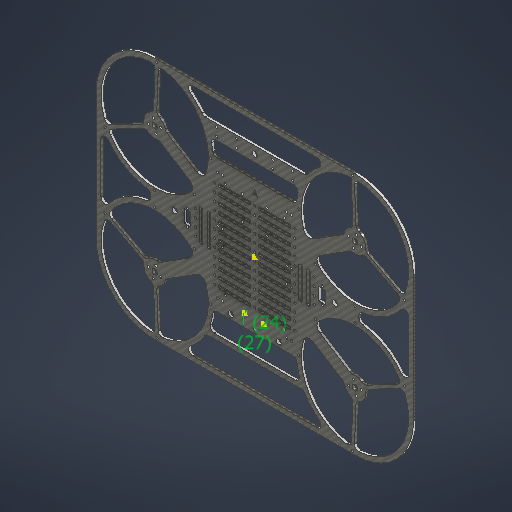
# Autodesk Inventor part: v3_bottom_carbon_fiber
Saved by Autodesk Inventor 2026 (Build 300175050, 175E)
## iProperties
Created: 2025-03-06
Part Number: v3_bottom_carbon_fiber
Material: Generic
Document SubType Name: Modeling
Designer: Bruno
Density: 1 g/cm^3
Appearance: Default
Author: Bruno
Autodesk Inventor part; units mm, degrees
ref_plane "YZ Plane" through (0, 0, 0) normal (1, 0, 0) x (0, 1, 0)
ref_plane "XZ Plane" through (0, 0, 0) normal (0, 1, 0) x (-1, 0, 0)
ref_plane "XY Plane" through (0, 0, 0) normal (0, 0, 1) x (1, 0, 0)
sketch "Sketch1" plane through (0, 0, 0) normal (0, 0, 1) x (1, 0, 0)
  line L0 (-125, 79) -> (125, 79)
  line L1 (-125, 79) -> (-125, -79)
  line L2 (-125, -79) -> (125, -79)
  line L3 (125, -79) -> (125, 79)
  line L4 (-234.9943, 0) -> (246.4628, 0)
  line L5 (0, 171.5298) -> (0, -171.5298)
  line L6 (52.1097, 83) -> (0, 83)
  line L7 (130, 6.1714) -> (130, 0)
  line L8 (198, 79) -> (198, 0)
  line L9 (125, 152) -> (0, 152)
  line L10 (52.1097, -83) -> (0, -83)
  line L11 (130, -6.1714) -> (130, 0)
  line L12 (198, -79) -> (198, 0)
  line L13 (125, -152) -> (0, -152)
  line L14 (125, 146) -> (0, 146)
  line L15 (192, 79) -> (192, 0)
  line L16 (125, -146) -> (0, -146)
  line L17 (192, -79) -> (192, 0)
  line L18 (-52.1097, 83) -> (0, 83)
  line L19 (-130, 6.1714) -> (-130, 0)
  line L20 (-198, 79) -> (-198, 0)
  line L21 (-125, 152) -> (0, 152)
  line L22 (-125, -152) -> (0, -152)
  line L23 (-52.1097, -83) -> (0, -83)
  line L24 (-198, -79) -> (-198, 0)
  line L25 (-130, -6.1714) -> (-130, 0)
  line L26 (-125, 146) -> (0, 146)
  line L27 (-192, 79) -> (-192, 0)
  line L28 (-125, -146) -> (0, -146)
  line L29 (-192, -79) -> (-192, 0)
  circle A0 centre (122.1995, 148.944) radius 1.5
  circle A1 centre (186.9735, 46.4534) radius 1.5
  circle A2 centre (125, 9) radius 1.5
  circle A3 centre (55, 79) radius 1.5
  circle A4 centre (75.5025, 29.5025) radius 1.5
  circle A5 centre (122.1995, -148.944) radius 1.5
  circle A6 centre (186.9735, -46.4534) radius 1.5
  circle A7 centre (125, -9) radius 1.5
  circle A8 centre (55, -79) radius 1.5
  circle A9 centre (75.5025, -29.5025) radius 1.5
  circle A10 centre (-122.1995, 148.944) radius 1.5
  circle A11 centre (-186.9735, 46.4534) radius 1.5
  circle A12 centre (-125, 9) radius 1.5
  circle A13 centre (-55, 79) radius 1.5
  circle A14 centre (-75.5025, 29.5025) radius 1.5
  circle A15 centre (-122.1995, -148.944) radius 1.5
  circle A16 centre (-55, -79) radius 1.5
  circle A17 centre (-75.5025, -29.5025) radius 1.5
  circle A18 centre (-125, -9) radius 1.5
  circle A19 centre (-186.9735, -46.4534) radius 1.5
  line L30 (-125, -79) -> (125, 79)
  line L31 (75.5025, 29.5025) -> (125, 79)
  line L32 (122.1995, 148.944) -> (125, 79)
  line L33 (125, 79) -> (186.9735, 46.4534)
  circle A20 centre (125, 79) radius 70
  circle A21 centre (125, 79) radius 13.5
  circle A22 centre (125, 79) radius 3.5
  circle A23 centre (125, 79) radius 8
  line L34 (120.0816, 66.4278) -> (73.0422, 36.6989)
  line L35 (111.5337, 79.9531) -> (64.4942, 50.2241)
  line L36 (126.4643, 92.4204) -> (124.3191, 145.9965)
  line L37 (135.8902, 71.0217) -> (183.3612, 46.0914)
  line L38 (122.4675, 92.2603) -> (120.3223, 145.8365)
  line L39 (137.7501, 74.5631) -> (185.221, 49.6328)
  circle A24 centre (125, -79) radius 13.5
  circle A25 centre (125, -79) radius 3.5
  line L40 (120.0816, -66.4278) -> (73.0422, -36.6989)
  line L41 (111.5337, -79.9531) -> (64.4942, -50.2241)
  line L42 (126.4643, -92.4204) -> (124.3191, -145.9965)
  line L43 (135.8902, -71.0217) -> (183.3612, -46.0914)
  line L44 (122.4675, -92.2603) -> (120.3223, -145.8365)
  line L45 (137.7501, -74.5631) -> (185.221, -49.6328)
  circle A26 centre (-125, 79) radius 13.5
  circle A27 centre (-125, 79) radius 3.5
  line L46 (-120.0816, 66.4278) -> (-73.0422, 36.6989)
  line L47 (-111.5337, 79.9531) -> (-64.4942, 50.2241)
  line L48 (-126.4643, 92.4204) -> (-124.3191, 145.9965)
  line L49 (-135.8902, 71.0217) -> (-183.3612, 46.0914)
  line L50 (-122.4675, 92.2603) -> (-120.3223, 145.8365)
  line L51 (-137.7501, 74.5631) -> (-185.221, 49.6328)
  circle A28 centre (-125, -79) radius 13.5
  circle A29 centre (-125, -79) radius 3.5
  line L52 (-137.7501, -74.5631) -> (-185.221, -49.6328)
  line L53 (-135.8902, -71.0217) -> (-183.3612, -46.0914)
  line L54 (-120.0816, -66.4278) -> (-73.0422, -36.6989)
  line L55 (-111.5337, -79.9531) -> (-64.4942, -50.2241)
  line L56 (-122.4675, -92.2603) -> (-120.3223, -145.8365)
  line L57 (-126.4643, -92.4204) -> (-124.3191, -145.9965)
  circle A30 centre (125, 79) radius 67
  circle A31 centre (125, 79) radius 73
  circle A32 centre (125, -79) radius 67
  circle A33 centre (125, -79) radius 73
  circle A34 centre (-125, 79) radius 67
  circle A35 centre (-125, 79) radius 73
  circle A36 centre (-125, -79) radius 67
  circle A37 centre (-125, -79) radius 73
  circle A38 centre (117.1959, 80.7597) radius 1.5
  line L58 (117.1959, 80.7597) -> (125, 79)
  circle A39 centre (123.2403, 71.1959) radius 1.5
  circle A40 centre (132.8041, 77.2403) radius 1.5
  circle A41 centre (126.7597, 86.8041) radius 1.5
  circle A42 centre (117.1959, -80.7597) radius 1.5
  circle A43 centre (123.2403, -71.1959) radius 1.5
  circle A44 centre (132.8041, -77.2403) radius 1.5
  circle A45 centre (126.7597, -86.8041) radius 1.5
  circle A46 centre (-117.1959, 80.7597) radius 1.5
  circle A47 centre (-123.2403, 71.1959) radius 1.5
  circle A48 centre (-132.8041, 77.2403) radius 1.5
  circle A49 centre (-126.7597, 86.8041) radius 1.5
  circle A50 centre (-117.1959, -80.7597) radius 1.5
  circle A51 centre (-126.7597, -86.8041) radius 1.5
  circle A52 centre (-123.2403, -71.1959) radius 1.5
  circle A53 centre (-132.8041, -77.2403) radius 1.5
  point P0 (0, 0)
  point P1 (-125, 0)
  point P2 (125, 0)
  point P3 (0, 79)
  point P4 (0, 0)
  point P5 (111.5337, 79.9531)
  point P6 (-111.5337, 79.9531)
  point P7 (-122.4675, 92.2603)
  point P8 (-137.7501, -74.5631)
  point P9 (-122.4675, -92.2603)
  point P10 (-111.5337, -79.9531)
  point P11 (111.5337, -79.9531)
  point P12 (122.4675, -92.2603)
  point P13 (137.7501, -74.5631)
  point P14 (73.0422, 36.6989)
  point P15 (115.6927, 140.8593)
  point P16 (122.3195, 145.9464)
  point P17 (122.3173, 146)
  point P18 (120, 141)
  point P19 (192, 50.0172)
  point P20 (192, -50.0172)
  point P21 (-125, 152)
  point P22 (-198, 79)
  point P23 (-198, -79)
  point P24 (-125, -152)
  point P25 (125, -152)
  point P26 (198, -79)
  point P27 (96.0172, 146)
  point P28 (-96.0172, 146)
  point P29 (52.1097, -83)
  point P30 (96.0172, -146)
  point P31 (-96.0172, -146)
  point P32 (-52.1097, -83)
  point P33 (-183.3612, 46.0914)
  point P34 (-119.6903, 140.9993)
  point P35 (-192, -50.0172)
  point P36 (-192, 50.0172)
  point P37 (-130, -6.1714)
  point P38 (-73.0422, -36.6989)
  point P39 (-120.3223, -145.8365)
  point P40 (-119.6903, -140.9993)
  point P41 (-185.221, -49.6328)
  point P42 (-183.3612, -46.0914)
  point P43 (64.4942, -50.2241)
  point P44 (73.0422, -36.6989)
  point P45 (124.3191, -145.9965)
  point P46 (120.3223, -145.8365)
  point P47 (124.4599, 92.4892)
  point P48 (68.363, 43.2054)
  point P49 (113.5881, 71.7877)
  dimension "d71" = 16
  dimension "d2" = 250
  dimension "d3" = 158
  dimension "d16" = 166
  dimension "d17" = 260
  dimension "d35" = 3
  dimension "d36" = 3
  dimension "d37" = 3
  dimension "d40" = 3
  dimension "d42" = 3
  dimension "d62" = 45
  dimension "d64" = 120
  dimension "d65" = 120
  dimension "d66" = 140
  dimension "d67" = 27
  dimension "d68" = 7
  dimension "d76" = 16
  dimension "d77" = 4
  dimension "d78" = 4
  dimension "d95" = 32.293
  dimension "d150" = 134
  dimension "d151" = 146
  dimension "d158" = 3
  dimension "d159" = 45
  dimension "d162" = 360
  dimension "d168" = 6
  constraints: 118 end point, 100 symmetric about line, 53 centre point, 31 point on circle, 14 coincident, 11 point on line, 7 perpendicular, 6 parallel, 6 tangent, 4 midpoint, 3 horizontal, 1 vertical, 51 other
  measures "d2" distance of L0.start L0.end
  measures "d3" distance of L2.end L0.end
  measures "d16" diameter of L6 L4
  measures "d17" diameter of L7 L5
  measures "d35" diameter of A0
  measures "d36" diameter of A1
  measures "d37" diameter of A2
  measures "d40" diameter of A3
  measures "d42" diameter of A4
  measures "d62" angle of L0 L31
  measures "d64" angle of L30 L33
  measures "d65" angle of L30 L32
  measures "d66" diameter of A20
  measures "d67" diameter of A21
  measures "d68" diameter of A22
  measures "d76" diameter of L34 L30
  measures "d77" diameter of L36 L32
  measures "d78" diameter of L37 L33
  measures "d95" angle of L30 L0
  measures "d150" diameter of A30
  measures "d151" diameter of A31
  measures "d158" diameter of A38
  measures "d159" angle of L30 L58
  measures "d168" radial gap between concentric circles of A31 A30
extrude "Extrusion1" add sketch "Sketch1" along normal blind 3 contours A27 L1 A26 L0 | L0 A26 L1 A27 | A26 L47 L0 | L0 L47 A34 L46 A26 | A34 L0 A13 A35 L1 A12 | L1 A12 A35 L27 A34 | L49 A34 L51 A26 | A34 L26 A35 L0 A13 | A26 L48 A34 L50 | A35 L0 L5 L4 L1 | L1 L4 L19 A35 | L27 A35 L26 A34 | A35 L18 L5 L0 | L4 L30 A37 L1 | L1 A37 L25 L4 | L27 L4 L20 A35 | L5 L6 A31 L0 | L0 A31 L30 L5 | A35 L21 L5 L26 | A37 L30 A36 L1 A18 | L1 A18 A36 L29 A37 | L30 A31 L3 L4 | L4 L3 A33 L2 L5 | L5 L2 A37 L30 | L29 A37 L24 L4 | A31 L14 A20 A3 L0 | L0 A3 A20 L30 A31 | L5 L9 A31 L14 | A37 L2 A16 A36 L30 | L4 L11 A33 L3 | L3 A31 L7 L4 | L5 L23 A37 L2 | L2 A33 L10 L5 | L30 A20 A4 A2 L3 A31 | L29 A36 L28 A37 | A31 L15 A20 A0 L14 | A36 L55 L2 A28 L30 | L30 A28 L54 A36 | A37 L28 A36 L2 A16 | A33 L17 A32 L3 A7 | L3 A7 A32 L2 A8 A33 | L3 A2 A20 A1 L15 A31 | L2 A8 A32 L16 A33 | A20 A3 L0 A30 L30 | L30 A30 L31 A4 A20 | A20 L14 L32 A30 L0 A3 | A20 A0 L32 L14 | A28 L2 A29 L30 | L30 A29 L1 A28 | L15 A31 L8 L4 | L4 L12 A33 L17 | L16 A33 L13 L5 | L5 L22 A37 L28 | A30 L35 L0 A21 L30 | L30 A21 L31 L34 A30 | A36 L53 A28 L52 | L32 A0 A20 L15 A30 L14 | L14 A30 L32 | L1 A29 L2 A28 | L2 L55 A28 | A33 L16 A32 L17 | A20 A4 L31 A30 L3 A2 | A21 L0 A23 L30 | L30 A23 L31 A21 | L57 A28 L56 A36 | A30 L36 A21 L32 | L32 A21 L38 A30 | L3 A30 L33 A1 A20 A2 | A20 A1 L33 A30 L15 | A23 L0 A22 L30 | L30 A22 L31 A23 | A21 L32 A23 A38 L0 | L0 L35 A21 | A21 L34 L31 | L31 A23 A39 L3 A21 | A21 L33 A23 A40 A41 L32 | A24 L2 A25 L3 | L3 A25 L2 A24 | A32 L45 A24 L43 | L40 A24 L2 L41 A32 | L2 A24 L41 | L44 A24 L42 A32 | A23 A38 L58 A22 L0 | L31 A22 L3 A23 A39 | A30 L33 A21 L39 | A23 A41 A40 L33 A22 L32 | L32 A22 L58 A38 A23 | L3 A23 L33 A21 | L37 A21 L33 A30 | L3 A22 L33 A23
fillet "Fillet1" radius 5 47 edges at (-130, 6.1714, 1.5) (-52.1097, 83, 1.5) (-135.8902, 71.0217, 1.5) (-122.4675, 92.2603, 1.5) (-126.4643, 92.4204, 1.5) (-137.7501, 74.5631, 1.5) (-137.7501, -74.5631, 1.5) (-135.8902, -71.0217, 1.5) (-126.4643, -92.4204, 1.5) (-122.4675, -92.2603, 1.5) (126.4643, -92.4204, 1.5) (122.4675, -92.2603, 1.5) (137.7501, -74.5631, 1.5) (135.8902, -71.0217, 1.5) (137.7501, 74.5631, 1.5) (135.8902, 71.0217, 1.5) (126.4643, 92.4204, 1.5) (122.4675, 92.2603, 1.5) (-120.3223, 145.8365, 1.5) (-183.3612, 46.0914, 1.5) (-185.221, 49.6328, 1.5) (-192, 50.0172, 1.5) (-96.0172, 146, 1.5) (-130, -6.1714, 1.5) (-192, -50.0172, 1.5) (-185.221, -49.6328, 1.5) (-183.3612, -46.0914, 1.5) (-120.3223, -145.8365, 1.5) (-96.0172, -146, 1.5) (-52.1097, -83, 1.5) (52.1097, -83, 1.5) (96.0172, -146, 1.5) (120.3223, -145.8365, 1.5) (124.3191, -145.9965, 1.5) (192, -50.0172, 1.5) (185.221, -49.6328, 1.5) (183.3612, -46.0914, 1.5) (130, -6.1714, 1.5) (130, 6.1714, 1.5) (192, 50.0172, 1.5) (185.221, 49.6328, 1.5) (183.3612, 46.0914, 1.5) (124.3191, 145.9965, 1.5) (96.0172, 146, 1.5) (52.1097, 83, 1.5) (-124.3191, 145.9965, 1.5) (-124.3191, -145.9965, 1.5)
fillet "Fillet2" radius 5 8 edges at (120.0816, 66.4278, 1.5) (111.5337, 79.9531, 1.5) (120.0816, -66.4278, 1.5) (111.5337, -79.9531, 1.5) (-111.5337, -79.9531, 1.5) (-120.0816, -66.4278, 1.5) (-111.5337, 79.9531, 1.5) (-120.0816, 66.4278, 1.5)
fillet "Fillet3" radius 8 8 edges at (64.4942, -50.2241, 1.5) (73.0422, -36.6989, 1.5) (64.4942, 50.2241, 1.5) (73.0422, 36.6989, 1.5) (-64.4942, 50.2241, 1.5) (-73.0422, 36.6989, 1.5) (-73.0422, -36.6989, 1.5) (-64.4942, -50.2241, 1.5)
sketch "Sketch2" plane through (0, 0, 3) normal (0, 0, 1) x (1, 0, 0)
  line L0 (-253.4929, 0) -> (253.4929, 0)
  line L1 (0, 210.0752) -> (0, -210.0752)
  line L2 (-46, -68) -> (46, -68)
  line L3 (46, -68) -> (46, -10)
  line L4 (46, -10) -> (-46, -10)
  line L5 (-46, -10) -> (-46, -68)
  circle A0 centre (-46, -68) radius 1.5
  circle A1 centre (46, -68) radius 1.5
  circle A2 centre (46, -10) radius 1.5
  circle A3 centre (-46, -10) radius 1.5
  line L6 (-47.521, -83) -> (47.521, -83) projected
  line L7 (-44, -53) -> (-6, -53)
  line L8 (-5, -54) -> (-5, -56)
  line L9 (-6, -57) -> (-44, -57)
  line L10 (-45, -56) -> (-45, -54)
  circle A4 centre (0, -55) radius 1.5
  line L11 (-59.788, -55) -> (59.788, -55)
  circle A5 centre (-50, -55) radius 1.5
  arc A6 (-45, -56) -> (-44, -57) centre (-44, -56) ccw
  arc A7 (-44, -53) -> (-45, -54) centre (-44, -54) ccw
  arc A8 (-6, -57) -> (-5, -56) centre (-6, -56) ccw
  arc A9 (-5, -54) -> (-6, -53) centre (-6, -54) ccw
  line L12 (44, -53) -> (6, -53)
  line L13 (5, -54) -> (5, -56)
  line L14 (6, -57) -> (44, -57)
  line L15 (45, -56) -> (45, -54)
  circle A10 centre (50, -55) radius 1.5
  arc A11 (44, -57) -> (45, -56) centre (44, -56) ccw
  arc A12 (45, -54) -> (44, -53) centre (44, -54) ccw
  arc A13 (5, -56) -> (6, -57) centre (6, -56) ccw
  arc A14 (6, -53) -> (5, -54) centre (6, -54) ccw
  circle A15 centre (-50, -45) radius 1.5
  line L16 (-45, -46) -> (-45, -44)
  arc A16 (-44, -43) -> (-45, -44) centre (-44, -44) ccw
  line L17 (-44, -43) -> (-6, -43)
  arc A17 (-45, -46) -> (-44, -47) centre (-44, -46) ccw
  line L18 (-6, -47) -> (-44, -47)
  arc A18 (-5, -44) -> (-6, -43) centre (-6, -44) ccw
  line L19 (-5, -44) -> (-5, -46)
  arc A19 (-6, -47) -> (-5, -46) centre (-6, -46) ccw
  circle A20 centre (0, -45) radius 1.5
  line L20 (5, -44) -> (5, -46)
  arc A21 (6, -43) -> (5, -44) centre (6, -44) ccw
  line L21 (44, -43) -> (6, -43)
  arc A22 (5, -46) -> (6, -47) centre (6, -46) ccw
  line L22 (6, -47) -> (44, -47)
  arc A23 (44, -47) -> (45, -46) centre (44, -46) ccw
  line L23 (45, -46) -> (45, -44)
  arc A24 (45, -44) -> (44, -43) centre (44, -44) ccw
  circle A25 centre (50, -45) radius 1.5
  circle A26 centre (-50, -35) radius 1.5
  line L24 (-45, -36) -> (-45, -34)
  arc A27 (-44, -33) -> (-45, -34) centre (-44, -34) ccw
  line L25 (-44, -33) -> (-6, -33)
  arc A28 (-45, -36) -> (-44, -37) centre (-44, -36) ccw
  line L26 (-6, -37) -> (-44, -37)
  arc A29 (-5, -34) -> (-6, -33) centre (-6, -34) ccw
  line L27 (-5, -34) -> (-5, -36)
  arc A30 (-6, -37) -> (-5, -36) centre (-6, -36) ccw
  circle A31 centre (0, -35) radius 1.5
  line L28 (5, -34) -> (5, -36)
  arc A32 (6, -33) -> (5, -34) centre (6, -34) ccw
  line L29 (44, -33) -> (6, -33)
  arc A33 (5, -36) -> (6, -37) centre (6, -36) ccw
  line L30 (6, -37) -> (44, -37)
  arc A34 (44, -37) -> (45, -36) centre (44, -36) ccw
  line L31 (45, -36) -> (45, -34)
  arc A35 (45, -34) -> (44, -33) centre (44, -34) ccw
  circle A36 centre (50, -35) radius 1.5
  circle A37 centre (-50, -25) radius 1.5
  line L32 (-45, -26) -> (-45, -24)
  arc A38 (-44, -23) -> (-45, -24) centre (-44, -24) ccw
  line L33 (-44, -23) -> (-6, -23)
  arc A39 (-45, -26) -> (-44, -27) centre (-44, -26) ccw
  line L34 (-6, -27) -> (-44, -27)
  arc A40 (-5, -24) -> (-6, -23) centre (-6, -24) ccw
  line L35 (-5, -24) -> (-5, -26)
  arc A41 (-6, -27) -> (-5, -26) centre (-6, -26) ccw
  circle A42 centre (0, -25) radius 1.5
  line L36 (5, -24) -> (5, -26)
  arc A43 (6, -23) -> (5, -24) centre (6, -24) ccw
  line L37 (44, -23) -> (6, -23)
  arc A44 (5, -26) -> (6, -27) centre (6, -26) ccw
  line L38 (6, -27) -> (44, -27)
  arc A45 (44, -27) -> (45, -26) centre (44, -26) ccw
  line L39 (45, -26) -> (45, -24)
  arc A46 (45, -24) -> (44, -23) centre (44, -24) ccw
  circle A47 centre (50, -25) radius 1.5
  circle A48 centre (-50, -15) radius 1.5
  line L40 (-45, -16) -> (-45, -14)
  arc A49 (-44, -13) -> (-45, -14) centre (-44, -14) ccw
  line L41 (-44, -13) -> (-6, -13)
  arc A50 (-45, -16) -> (-44, -17) centre (-44, -16) ccw
  line L42 (-6, -17) -> (-44, -17)
  arc A51 (-5, -14) -> (-6, -13) centre (-6, -14) ccw
  line L43 (-5, -14) -> (-5, -16)
  arc A52 (-6, -17) -> (-5, -16) centre (-6, -16) ccw
  circle A53 centre (0, -15) radius 1.5
  line L44 (5, -14) -> (5, -16)
  arc A54 (6, -13) -> (5, -14) centre (6, -14) ccw
  line L45 (44, -13) -> (6, -13)
  arc A55 (5, -16) -> (6, -17) centre (6, -16) ccw
  line L46 (6, -17) -> (44, -17)
  arc A56 (44, -17) -> (45, -16) centre (44, -16) ccw
  line L47 (45, -16) -> (45, -14)
  arc A57 (45, -14) -> (44, -13) centre (44, -14) ccw
  circle A58 centre (50, -15) radius 1.5
  circle A59 centre (-50, -5) radius 1.5
  line L48 (-45, -6) -> (-45, -4)
  arc A60 (-44, -3) -> (-45, -4) centre (-44, -4) ccw
  line L49 (-44, -3) -> (-6, -3)
  arc A61 (-45, -6) -> (-44, -7) centre (-44, -6) ccw
  line L50 (-6, -7) -> (-44, -7)
  arc A62 (-5, -4) -> (-6, -3) centre (-6, -4) ccw
  line L51 (-5, -4) -> (-5, -6)
  arc A63 (-6, -7) -> (-5, -6) centre (-6, -6) ccw
  circle A64 centre (0, -5) radius 1.5
  line L52 (5, -4) -> (5, -6)
  arc A65 (6, -3) -> (5, -4) centre (6, -4) ccw
  line L53 (44, -3) -> (6, -3)
  arc A66 (5, -6) -> (6, -7) centre (6, -6) ccw
  line L54 (6, -7) -> (44, -7)
  arc A67 (44, -7) -> (45, -6) centre (44, -6) ccw
  line L55 (45, -6) -> (45, -4)
  arc A68 (45, -4) -> (44, -3) centre (44, -4) ccw
  circle A69 centre (50, -5) radius 1.5
  circle A70 centre (-50, 5) radius 1.5
  line L56 (-45, 4) -> (-45, 6)
  arc A71 (-44, 7) -> (-45, 6) centre (-44, 6) ccw
  line L57 (-44, 7) -> (-6, 7)
  arc A72 (-45, 4) -> (-44, 3) centre (-44, 4) ccw
  line L58 (-6, 3) -> (-44, 3)
  arc A73 (-5, 6) -> (-6, 7) centre (-6, 6) ccw
  line L59 (-5, 6) -> (-5, 4)
  arc A74 (-6, 3) -> (-5, 4) centre (-6, 4) ccw
  circle A75 centre (0, 5) radius 1.5
  line L60 (5, 6) -> (5, 4)
  arc A76 (6, 7) -> (5, 6) centre (6, 6) ccw
  line L61 (44, 7) -> (6, 7)
  arc A77 (5, 4) -> (6, 3) centre (6, 4) ccw
  line L62 (6, 3) -> (44, 3)
  arc A78 (44, 3) -> (45, 4) centre (44, 4) ccw
  line L63 (45, 4) -> (45, 6)
  arc A79 (45, 6) -> (44, 7) centre (44, 6) ccw
  circle A80 centre (50, 5) radius 1.5
  circle A81 centre (-50, 15) radius 1.5
  line L64 (-45, 14) -> (-45, 16)
  arc A82 (-44, 17) -> (-45, 16) centre (-44, 16) ccw
  line L65 (-44, 17) -> (-6, 17)
  arc A83 (-45, 14) -> (-44, 13) centre (-44, 14) ccw
  line L66 (-6, 13) -> (-44, 13)
  arc A84 (-5, 16) -> (-6, 17) centre (-6, 16) ccw
  line L67 (-5, 16) -> (-5, 14)
  arc A85 (-6, 13) -> (-5, 14) centre (-6, 14) ccw
  circle A86 centre (0, 15) radius 1.5
  line L68 (5, 16) -> (5, 14)
  arc A87 (6, 17) -> (5, 16) centre (6, 16) ccw
  line L69 (44, 17) -> (6, 17)
  arc A88 (5, 14) -> (6, 13) centre (6, 14) ccw
  line L70 (6, 13) -> (44, 13)
  arc A89 (44, 13) -> (45, 14) centre (44, 14) ccw
  line L71 (45, 14) -> (45, 16)
  arc A90 (45, 16) -> (44, 17) centre (44, 16) ccw
  circle A91 centre (50, 15) radius 1.5
  circle A92 centre (-50, 25) radius 1.5
  line L72 (-45, 24) -> (-45, 26)
  arc A93 (-44, 27) -> (-45, 26) centre (-44, 26) ccw
  line L73 (-44, 27) -> (-6, 27)
  arc A94 (-45, 24) -> (-44, 23) centre (-44, 24) ccw
  line L74 (-6, 23) -> (-44, 23)
  arc A95 (-5, 26) -> (-6, 27) centre (-6, 26) ccw
  line L75 (-5, 26) -> (-5, 24)
  arc A96 (-6, 23) -> (-5, 24) centre (-6, 24) ccw
  circle A97 centre (0, 25) radius 1.5
  line L76 (5, 26) -> (5, 24)
  arc A98 (6, 27) -> (5, 26) centre (6, 26) ccw
  line L77 (44, 27) -> (6, 27)
  arc A99 (5, 24) -> (6, 23) centre (6, 24) ccw
  line L78 (6, 23) -> (44, 23)
  arc A100 (44, 23) -> (45, 24) centre (44, 24) ccw
  line L79 (45, 24) -> (45, 26)
  arc A101 (45, 26) -> (44, 27) centre (44, 26) ccw
  circle A102 centre (50, 25) radius 1.5
  circle A103 centre (-50, 35) radius 1.5
  line L80 (-45, 34) -> (-45, 36)
  arc A104 (-44, 37) -> (-45, 36) centre (-44, 36) ccw
  line L81 (-44, 37) -> (-6, 37)
  arc A105 (-45, 34) -> (-44, 33) centre (-44, 34) ccw
  line L82 (-6, 33) -> (-44, 33)
  arc A106 (-5, 36) -> (-6, 37) centre (-6, 36) ccw
  line L83 (-5, 36) -> (-5, 34)
  arc A107 (-6, 33) -> (-5, 34) centre (-6, 34) ccw
  circle A108 centre (0, 35) radius 1.5
  line L84 (5, 36) -> (5, 34)
  arc A109 (6, 37) -> (5, 36) centre (6, 36) ccw
  line L85 (44, 37) -> (6, 37)
  arc A110 (5, 34) -> (6, 33) centre (6, 34) ccw
  line L86 (6, 33) -> (44, 33)
  arc A111 (44, 33) -> (45, 34) centre (44, 34) ccw
  line L87 (45, 34) -> (45, 36)
  arc A112 (45, 36) -> (44, 37) centre (44, 36) ccw
  circle A113 centre (50, 35) radius 1.5
  circle A114 centre (-50, 45) radius 1.5
  line L88 (-45, 44) -> (-45, 46)
  arc A115 (-44, 47) -> (-45, 46) centre (-44, 46) ccw
  line L89 (-44, 47) -> (-6, 47)
  arc A116 (-45, 44) -> (-44, 43) centre (-44, 44) ccw
  line L90 (-6, 43) -> (-44, 43)
  arc A117 (-5, 46) -> (-6, 47) centre (-6, 46) ccw
  line L91 (-5, 46) -> (-5, 44)
  arc A118 (-6, 43) -> (-5, 44) centre (-6, 44) ccw
  circle A119 centre (0, 45) radius 1.5
  line L92 (5, 46) -> (5, 44)
  arc A120 (6, 47) -> (5, 46) centre (6, 46) ccw
  line L93 (44, 47) -> (6, 47)
  arc A121 (5, 44) -> (6, 43) centre (6, 44) ccw
  line L94 (6, 43) -> (44, 43)
  arc A122 (44, 43) -> (45, 44) centre (44, 44) ccw
  line L95 (45, 44) -> (45, 46)
  arc A123 (45, 46) -> (44, 47) centre (44, 46) ccw
  circle A124 centre (50, 45) radius 1.5
  circle A125 centre (-50, 55) radius 1.5
  line L96 (-45, 54) -> (-45, 56)
  arc A126 (-44, 57) -> (-45, 56) centre (-44, 56) ccw
  line L97 (-44, 57) -> (-6, 57)
  arc A127 (-45, 54) -> (-44, 53) centre (-44, 54) ccw
  line L98 (-6, 53) -> (-44, 53)
  arc A128 (-5, 56) -> (-6, 57) centre (-6, 56) ccw
  line L99 (-5, 56) -> (-5, 54)
  arc A129 (-6, 53) -> (-5, 54) centre (-6, 54) ccw
  circle A130 centre (0, 55) radius 1.5
  line L100 (5, 56) -> (5, 54)
  arc A131 (6, 57) -> (5, 56) centre (6, 56) ccw
  line L101 (44, 57) -> (6, 57)
  arc A132 (5, 54) -> (6, 53) centre (6, 54) ccw
  line L102 (6, 53) -> (44, 53)
  arc A133 (44, 53) -> (45, 54) centre (44, 54) ccw
  line L103 (45, 54) -> (45, 56)
  arc A134 (45, 56) -> (44, 57) centre (44, 56) ccw
  circle A135 centre (50, 55) radius 1.5
  line L104 (0, 73) -> (-3.5, 65)
  line L105 (-3.5, 65) -> (0, 67)
  line L106 (0, 73) -> (3.5, 65)
  line L107 (3.5, 65) -> (0, 67)
  line L108 (-62, 19) -> (-62, -19)
  line L109 (-58, 20) -> (-56, 20)
  line L110 (-55, 19) -> (-55, -19)
  line L111 (-56, -20) -> (-58, -20)
  line L112 (-59, -19) -> (-59, 19)
  arc A136 (-55, 19) -> (-56, 20) centre (-56, 19) ccw
  arc A137 (-58, 20) -> (-59, 19) centre (-58, 19) ccw
  arc A138 (-59, -19) -> (-58, -20) centre (-58, -19) ccw
  arc A139 (-56, -20) -> (-55, -19) centre (-56, -19) ccw
  circle A140 centre (-74, -15) radius 1.5
  circle A141 centre (-74, -5) radius 1.5
  circle A142 centre (-74, 5) radius 1.5
  circle A143 centre (-74, 15) radius 1.5
  line L113 (-66, 20) -> (-68, 20)
  line L114 (-69, 19) -> (-69, -19)
  line L115 (-68, -20) -> (-66, -20)
  line L116 (-65, -19) -> (-65, 19)
  arc A144 (-68, 20) -> (-69, 19) centre (-68, 19) ccw
  arc A145 (-65, 19) -> (-66, 20) centre (-66, 19) ccw
  arc A146 (-66, -20) -> (-65, -19) centre (-66, -19) ccw
  arc A147 (-69, -19) -> (-68, -20) centre (-68, -19) ccw
  line L117 (58, 20) -> (56, 20)
  line L118 (55, 19) -> (55, -19)
  line L119 (56, -20) -> (58, -20)
  line L120 (59, -19) -> (59, 19)
  arc A148 (56, 20) -> (55, 19) centre (56, 19) ccw
  arc A149 (59, 19) -> (58, 20) centre (58, 19) ccw
  arc A150 (58, -20) -> (59, -19) centre (58, -19) ccw
  arc A151 (55, -19) -> (56, -20) centre (56, -19) ccw
  line L121 (69, 19) -> (69, -19)
  arc A152 (69, 19) -> (68, 20) centre (68, 19) ccw
  line L122 (66, 20) -> (68, 20)
  arc A153 (66, 20) -> (65, 19) centre (66, 19) ccw
  line L123 (65, -19) -> (65, 19)
  circle A154 centre (74, 15) radius 1.5
  circle A155 centre (74, 5) radius 1.5
  circle A156 centre (74, -5) radius 1.5
  circle A157 centre (74, -15) radius 1.5
  line L124 (68, -20) -> (66, -20)
  arc A158 (65, -19) -> (66, -20) centre (66, -19) ccw
  arc A159 (68, -20) -> (69, -19) centre (68, -19) ccw
  circle A160 centre (-40, -68) radius 1.5
  circle A161 centre (40, -68) radius 1.5
  circle A162 centre (-40, -10) radius 1.5
  circle A163 centre (40, -10) radius 1.5
  circle A164 centre (-46, 68) radius 1.5
  circle A165 centre (46, 68) radius 1.5
  circle A166 centre (46, 10) radius 1.5
  circle A167 centre (-46, 10) radius 1.5
  circle A168 centre (-40, 68) radius 1.5
  circle A169 centre (40, 68) radius 1.5
  circle A170 centre (-40, 10) radius 1.5
  circle A171 centre (40, 10) radius 1.5
  circle A172 centre (-100, 0) radius 3.25
  line L125 (-101.7321, 2.75) -> (-98.2679, 2.75)
  circle A173 centre (-30, -77) radius 3.25
  line L126 (-31.7321, -74.25) -> (-28.2679, -74.25)
  circle A174 centre (0, -79) radius 1.5
  circle A175 centre (-12, -67) radius 1.5
  circle A176 centre (100, 0) radius 3.25
  line L127 (101.7321, 2.75) -> (98.2679, 2.75)
  circle A177 centre (30, -77) radius 3.25
  line L128 (31.7321, -74.25) -> (28.2679, -74.25)
  circle A178 centre (12, -67) radius 1.5
  line L129 (-88.1, 7.8) -> (-80, 7.8)
  line L130 (-80, 7.8) -> (-80, -7.8)
  line L131 (-80, -7.8) -> (-88.1, -7.8)
  line L132 (-88.1, -7.8) -> (-88.1, 7.8)
  line L133 (-84.05, 25.3536) -> (-84.05, -25.3536)
  circle A179 centre (-84.05, 10.25) radius 1.5
  line L134 (-84.05, -25.3536) -> (-84.05, 25.3536)
  circle A180 centre (-84.05, -10.25) radius 1.5
  line L135 (88.1, 7.8) -> (80, 7.8)
  line L136 (80, 7.8) -> (80, -7.8)
  line L137 (80, -7.8) -> (88.1, -7.8)
  line L138 (88.1, -7.8) -> (88.1, 7.8)
  circle A181 centre (84.05, 10.25) radius 1.5
  circle A182 centre (84.05, -10.25) radius 1.5
  line L139 (-24.2593, 45) -> (24.2593, 45)
  circle A183 centre (-15.25, 60.25) radius 1.5
  circle A184 centre (-15.25, 29.75) radius 1.5
  circle A185 centre (15.25, 60.25) radius 1.5
  circle A186 centre (15.25, 29.75) radius 1.5
  circle A187 centre (-37, -60) radius 1.5
  circle A188 centre (37, -60) radius 1.5
  circle A189 centre (-37, 60) radius 1.5
  circle A190 centre (37, 60) radius 1.5
  point P0 (0, 0)
  point P1 (0, 0)
  point P2 (-5, -57)
  point P3 (-45, -57)
  point P4 (-5, -55)
  point P5 (-45, -47)
  point P6 (-5, -47)
  point P7 (-5, -45)
  point P8 (-45, -37)
  point P9 (-5, -37)
  point P10 (-5, -35)
  point P11 (-45, -27)
  point P12 (-5, -27)
  point P13 (-5, -25)
  point P14 (-45, -17)
  point P15 (-5, -17)
  point P16 (-5, -15)
  point P17 (-45, -7)
  point P18 (-5, -7)
  point P19 (-5, -5)
  point P20 (-45, 3)
  point P21 (-5, 3)
  point P22 (-5, 5)
  point P23 (-45, 13)
  point P24 (-5, 13)
  point P25 (-5, 15)
  point P26 (-45, 23)
  point P27 (-5, 23)
  point P28 (-5, 25)
  point P29 (-45, 33)
  point P30 (-5, 33)
  point P31 (-5, 35)
  point P32 (-45, 43)
  point P33 (-5, 43)
  point P34 (-5, 45)
  point P35 (-45, 53)
  point P36 (-5, 53)
  point P37 (-5, 55)
  point P38 (-62, 0)
  point P39 (-59, 20)
  point P40 (-55, -20)
  point P41 (-55, 20)
  point P42 (-55, 0)
  point P43 (0, -68)
  point P44 (-88.1, 0)
  point P45 (-84.05, 0)
  point P46 (-84.05, 7.8)
  point P47 (0, 45)
  dimension "d45" = 92
  dimension "d46" = 58
  dimension "d47" = 3
  dimension "d48" = 3
  dimension "d49" = 3
  dimension "d50" = 3
  dimension "d55" = 15
  dimension "d79" = 3
  dimension "d80" = 4
  dimension "d81" = 40
  dimension "d82" = 10
  dimension "d83" = 3
  dimension "d86" = 1
  dimension "d89" = 10
  dimension "d94" = 6
  dimension "d96" = 100
  dimension "d97" = 7
  dimension "d98" = 6
  dimension "d99" = 8
  dimension "d100" = 10
  dimension "d101" = 62
  dimension "d102" = 4
  dimension "d103" = 6
  dimension "d104" = 40
  dimension "d105" = 1
  dimension "d106" = 3
  dimension "d107" = 3
  dimension "d108" = 6
  dimension "d109" = 6
  dimension "d110" = 3
  dimension "d111" = 3
  dimension "d112" = 6
  dimension "d113" = 6
  dimension "d133" = 6.5
  dimension "d134" = 200
  dimension "d135" = 6
  dimension "d136" = 6.5
  dimension "d137" = 6
  dimension "d138" = 60
  dimension "d139" = 6
  dimension "d140" = 3
  dimension "d141" = 3
  dimension "d142" = 24
  dimension "d143" = 24
  dimension "d144" = 24
  dimension "d145" = 8.1
  dimension "d146" = 15.6
  dimension "d147" = 160
  dimension "d148" = 3
  dimension "d149" = 20.5
  dimension "d164" = 3
  dimension "d165" = 30.5
  dimension "d166" = 30.5
  dimension "d167" = 45
  dimension "d169" = 3
  dimension "d170" = 74
  dimension "d171" = 120
  constraints: 330 vertical alignment, 276 end point, 232 point on circle, 191 centre point, 152 equal radius, 68 point on line, 58 horizontal alignment, 52 parallel, 44 collinear, 30 symmetric about line, 16 tangent, 10 midpoint, 9 horizontal, 5 coincident, 4 perpendicular, 2 vertical, 30 other
  measures "d45" distance of L2.start L2.end
  measures "d46" distance of L4.end L2.start
  measures "d47" diameter of A3
  measures "d48" diameter of A0
  measures "d49" diameter of A1
  measures "d50" diameter of A2
  measures "d55" distance between parallel lines of L6 L2
  measures "d79" diameter of A4
  measures "d80" distance between parallel lines of L9 L7
  measures "d81" distance of point (-5, -57) point (-45, -57)
  measures "d83" diameter of A5
  measures "d86" radius of A6
  measures "d89" distance of A5.centre A15.centre
  measures "d94" diameter of L58 L0
  measures "d98" distance of L104.start L105.end
  measures "d99" vertical distance of L104.end L104.start
  measures "d100" distance from line of L101 L105.end
  measures "d101" distance of the line from the sketch origin of L108
  measures "d102" distance of point (-59, 20) point (-55, 20)
  measures "d103" diameter of L112 L108
  measures "d104" distance of point (-55, 20) point (-55, -20)
  measures "d105" radius of A136
  measures "d106" diameter of A160
  measures "d107" diameter of A161
  measures "d108" distance of L2.start A160.centre
  measures "d109" distance of L2.end A161.centre
  measures "d110" diameter of A162
  measures "d111" diameter of A163
  measures "d112" distance of L4.end A162.centre
  measures "d113" distance of L3.end A163.centre
  measures "d133" diameter of A172
  measures "d136" diameter of A173
  measures "d139" distance from line of L6 A173.centre
  measures "d140" diameter of A174
  measures "d141" diameter of A175
  measures "d142" distance of A4.centre A174.centre
  measures "d144" diameter of A175.centre L11
  measures "d145" distance of L129.start L129.end
  measures "d146" distance of L129.end L130.end
  measures "d148" diameter of A179
  measures "d149" diameter of A179.centre L0
  measures "d164" diameter of A183
  measures "d165" diameter of A183.centre L139
  measures "d167" distance between parallel lines of L0 L139
  measures "d169" diameter of A187
  measures "d171" diameter of A187.centre L0
extrude "Extrusion2" cut sketch "Sketch2" against normal through all contours A172 L125 L0 | A179 L133 | L133 A179 | L91 A118 L90 A116 L88 A115 L89 A117 | L105 L104 L1 | L1 L106 L107 | A130 L1 | L1 A130 | L92 A120 L93 A123 L95 A122 L94 A121 | A119 L139 L1 | L1 L139 A119 | A108 L1 | L1 A108 | A97 L1 | L1 A97 | A86 L1 | L1 A86 | A75 L1 | L1 A75 | A176 L127 L0 | L0 A176 | L136 L135 L138 L0 | L0 L138 L137 L136 | L123 A153 L122 A152 L121 L0 | L0 L121 A159 L124 A158 L123 | L118 A148 L117 A149 L120 L0 | L0 L120 A150 L119 A151 L118 | A10 L11 | L11 A10 | A174 L1 | L1 A174 | A5 L11 | L11 A5 | A64 L1 | L1 A64 | L112 A137 L109 A136 L110 L0 | L0 L110 A139 L111 A138 L112 | L114 A144 L113 A145 L116 L0 | L0 L116 A146 L115 A147 L114 | A180 L133 | L133 A180 | L132 L129 L133 L0 | L0 L133 L131 L132 | L0 A172 | L133 L129 L130 L0 | L0 L130 L131 L133 | A53 L1 | L1 A53 | A163 L4 | L4 A163 | A162 L4 | L4 A162 | A42 L1 | L1 A42 | A2 L3 L4 | L4 L3 A2 | A3 L5 L4 | L4 L5 A3 | A31 L1 | L1 A31 | A1 L2 L3 | L3 L2 A1 | L15 A11 L14 A13 L13 L11 | L11 L13 A14 L12 A12 L15 | A0 L2 L5 | L5 L2 A0 | L11 L8 A8 L9 A6 L10 | L10 A7 L7 A9 L8 L11 | L139 A119 L1 | L1 A119 L139 | A20 L1 | L1 A20 | A161 L2 | L2 A161 | L11 L1 A4 | A4 L1 L11 | A160 L2 | L2 A160 | L11 L1 A4 | A4 L1 L11 | A178 L2 | L2 A178 | A175 L2 | L2 A175 | A15 | L16 A16 L17 A18 L19 A19 L18 A17 | A21 L21 A24 L23 A23 L22 A22 L20 | A25 | A26 | L24 A27 L25 A29 L27 A30 L26 A28 | A32 L29 A35 L31 A34 L30 A33 L28 | A36 | A37 | L32 A38 L33 A40 L35 A41 L34 A39 | A43 L37 A46 L39 A45 L38 A44 L36 | A47 | A48 | L40 A49 L41 A51 L43 A52 L42 A50 | A54 L45 A57 L47 A56 L46 A55 L44 | A58 | A59 | L48 A60 L49 A62 L51 A63 L50 A61 | A65 L53 A68 L55 A67 L54 A66 L52 | A69 | A70 | L56 A71 L57 A73 L59 A74 L58 A72 | A76 L61 A79 L63 A78 L62 A77 L60 | A80 | A81 | L64 A82 L65 A84 L67 A85 L66 A83 | A87 L69 A90 L71 A89 L70 A88 L68 | A91 | A92 | L72 A93 L73 A95 L75 A96 L74 A94 | A98 L77 A101 L79 A100 L78 A99 L76 | A102 | A103 | L80 A104 L81 A106 L83 A107 L82 A105 | A109 L85 A112 L87 A111 L86 A110 L84 | A113 | A114 | A124 | A125 | L96 A126 L97 A128 L99 A129 L98 A127 | A131 L101 A134 L103 A133 L102 A132 L100 | A135 | A140 | A141 | A142 | A143 | A154 | A155 | A156 | A157 | A164 | A165 | A166 | A167 | A168 | A169 | A170 | A171 | A173 L126 | A177 L128 | A181 | A182 | A183 | A184 | A185 | A186 | A187 | A188 | A189 | A190 picked at (-30.526, -76.5114) picked at (30.959, -77.519)
sketch "Sketch5" plane through (0, 0, 3) normal (0, 0, 1) x (1, 0, 0)
  line L0 (-64.6013, 120) -> (64.6013, 120)
  line L1 (-55.718, 102) -> (55.718, 102)
  line L2 (-58.0075, -108) -> (58.0075, -108)
  line L3 (-60.9375, -114) -> (62.5778, -114)
  line L4 (-47.521, -83) -> (47.521, -83) projected
  line L5 (-77.6714, 146) -> (77.6714, 146) projected
  arc A0 (-52.4876, 87.4231) -> (-80.7052, 137.0256) centre (-125, 79) ccw projected
  arc A1 (80.7052, 137.0256) -> (52.4876, 87.4231) centre (125, 79) ccw projected
  arc A2 (-80.7052, -137.0256) -> (-52.4876, -87.4231) centre (-125, -79) ccw projected
  arc A3 (52.4876, -87.4231) -> (80.7052, -137.0256) centre (125, -79) ccw projected
  point P0 (0, 0)
  point P1 (60.9375, -114)
  dimension "d114" = 6
  dimension "d115" = 25
  dimension "d116" = 18
  dimension "d117" = 26
  constraints: 8 end point, 6 point on circle, 2 horizontal, 2 parallel, 2 other
  measures "d114" distance between parallel lines of L3 L2
  measures "d115" distance between parallel lines of L4 L2
  measures "d116" distance between parallel lines of L1 L0
  measures "d117" distance between parallel lines of L5 L0
extrude "Extrusion4" add sketch "Sketch5" against normal up to surface (3 mm away)
fillet "Fillet4" radius 5 8 edges at (-55.718, 102, 1.5) (55.718, 102, 1.5) (64.6013, 120, 1.5) (-64.6013, 120, 1.5) (-60.9375, -114, 1.5) (-58.0075, -108, 1.5) (58.0075, -108, 1.5) (60.9375, -114, 1.5)
sketch "Sketch6" plane through (0, 0, 3) normal (0, 0, 1) x (1, 0, 0)
  line L0 (62.0079, 120) -> (-62.0079, 120) projected
  line L1 (-49.1053, 102) -> (49.1053, 102) projected
  line L2 (0, 120) -> (0, 102)
  line L3 (-85.715, 111) -> (85.715, 111)
  circle A0 centre (-47.5, 106) radius 1.5
  circle A1 centre (-47.5, 116) radius 1.5
  line L4 (-47.5, 106) -> (-47.5, 116)
  circle A2 centre (-22.5, 106) radius 1.5
  circle A3 centre (-22.5, 116) radius 1.5
  line L5 (-22.5, 106) -> (-22.5, 116)
  circle A4 centre (47.5, 106) radius 1.5
  circle A5 centre (47.5, 116) radius 1.5
  circle A6 centre (22.5, 106) radius 1.5
  circle A7 centre (22.5, 116) radius 1.5
  circle A8 centre (0, 111) radius 3.2
  point P0 (0, 0)
  point P1 (76.6872, 130)
  point P2 (-76.6872, 130)
  point P3 (-47.7504, 96)
  point P4 (47.7504, 96)
  point P5 (60.5021, 114)
  point P6 (-60.5021, 114)
  point P7 (63.079, 114)
  point P8 (-63.079, 114)
  point P9 (-54.2733, 96)
  point P10 (54.2733, 96)
  point P11 (62.5544, 115)
  point P12 (-62.5544, 115)
  point P13 (-53.547, 97)
  point P14 (53.547, 97)
  point P15 (-62.0079, 120)
  point P16 (49.1053, 102)
  dimension "d121" = 3
  dimension "d122" = 10
  dimension "d123" = 95
  dimension "d127" = 3
  dimension "d128" = 10
  dimension "d131" = 45
  dimension "d132" = 6.4
  constraints: 9 centre point, 8 end point, 6 symmetric about line, 2 midpoint, 2 vertical, 1 coincident, 1 horizontal, 10 other
  measures "d121" diameter of A0
  measures "d122" diameter of L4.start L3
  measures "d123" diameter of L4.start L2
  measures "d127" diameter of A2
  measures "d128" diameter of L5.start L3
  measures "d131" diameter of L5.start L2
  measures "d132" diameter of A8
extrude "Extrusion5" cut sketch "Sketch6" against normal blind 10
sketch "Sketch7" plane through (0, 0, 3) normal (0, 0, 1) x (1, 0, 0)
  circle A0 centre (-12, -67) radius 1.5 projected
  circle A1 centre (12, -67) radius 1.5 projected
  point P0 (0, 0)
  dimension "d172" = 27
sketch "Sketch8" plane through (0, 0, 3) normal (0, 0, 1) x (1, 0, 0)
  circle A0 centre (12, -67) radius 1.5 projected
  circle A1 centre (-12, -67) radius 1.5 projected
  point P0 (0, 0)
  dimension "d173" = 24
  measures "d173" distance of A0.centre A1.centre
sketch "Sketch3" plane through (0, 0, 0) normal (0, 0, -1) x (-1, 0, 0)
  line L0 (124, -100) -> (-124, -100)
  line L1 (-124, -100) -> (-124, 100)
  line L2 (-124, 100) -> (124, 100)
  line L3 (124, 100) -> (124, -100)
  line L4 (124, -100) -> (-124, 100)
  line L5 (204, -160) -> (-204, -160)
  line L6 (-204, -160) -> (-204, 160)
  line L7 (-204, 160) -> (204, 160)
  line L8 (204, 160) -> (204, -160)
  line L9 (-204, -160) -> (204, 160)
  point P0 (0, 0)
  point P1 (0, 0)
  dimension "d56" = 200
  dimension "d57" = 248
  dimension "d58" = 60
  dimension "d59" = 80
  constraints: 20 end point, 4 parallel, 2 horizontal, 2 midpoint, 2 perpendicular, 1 coincident
  measures "d56" distance of L2.end L0.start
  measures "d57" distance of L0.start L0.end
  measures "d58" distance between parallel lines of L0 L5
  measures "d59" distance between parallel lines of L8 L3
body "Solid1"
